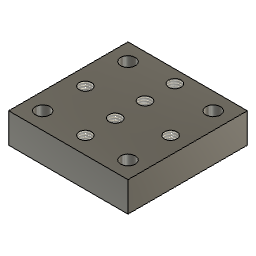
Dilution Attachment 28x28mm v2 (Autodesk Fusion 360 design; units mm, degrees)
Autodesk Fusion 360 part; units mm, degrees
note: some values were not read from the file. Set by a fixed rule: the direction of a hole.
sketch "Sketch1" plane through (0, 0, 0) normal (0, 0, 1) x (1, 0, 0)
  line L0 (0, 28) -> (28, 28)
  line L1 (28, 28) -> (28, 0)
  line L2 (28, 0) -> (0, 0)
  line L3 (0, 0) -> (0, 28)
  dimension "d1" = 28
  dimension "d2" = 28
  dimension "d13" = 28
  dimension "d14" = 28
  constraint horizontal L0
  constraint vertical L1
  constraint horizontal L2
  constraint vertical L3
  measures "d1" distance of L0.start L0.end
  measures "d2" distance of L0.start L2.end
  measures "d13" distance of L0.end L1.end
  measures "d14" distance of L1.end L2.end
sketch "Sketch2" plane through (0, 0, 0) normal (0, 0, 1) x (1, 0, 0)
  circle A0 centre (4, 24) radius 1.5
  circle A1 centre (4, 4) radius 1.5
  circle A2 centre (24, 4) radius 1.5
  circle A3 centre (24, 24) radius 1.5
  circle A4 centre (4, 14) radius 1.5
  circle A5 centre (14, 25) radius 1.5
  circle A6 centre (14, 18) radius 1.5
  circle A7 centre (14, 4) radius 1.5
  circle A8 centre (24, 14) radius 1.5
  circle A9 centre (14, 11) radius 1.5
  dimension "d15" = 3
  dimension "d16" = 3
  dimension "d17" = 3
  dimension "d18" = 3
  dimension "d19" = 3
  dimension "d20" = 3
  dimension "d21" = 3
  dimension "d22" = 3
  dimension "d23" = 3
  dimension "d24" = 3
  dimension "d25" = 10
  dimension "d26" = 10
  dimension "d27" = 10
  dimension "d28" = 10
  dimension "d29" = 10
  dimension "d30" = 10
  dimension "d31" = 7
  dimension "d32" = 7
  dimension "d33" = 7
  measures "d15" diameter of A0
  measures "d16" diameter of A5
  measures "d17" diameter of A3
  measures "d18" diameter of A6
  measures "d19" diameter of A4
  measures "d20" diameter of A8
  measures "d21" diameter of A9
  measures "d22" diameter of A7
  measures "d23" diameter of A2
  measures "d24" diameter of A1
  measures "d25" distance of A0.centre A4.centre
  measures "d26" distance of A1.centre A4.centre
  measures "d27" distance of A1.centre A7.centre
  measures "d28" distance of A2.centre A7.centre
  measures "d29" distance of A2.centre A8.centre
  measures "d30" distance of A3.centre A8.centre
  measures "d31" distance of A5.centre A6.centre
  measures "d32" distance of A6.centre A9.centre
  measures "d33" distance of A7.centre A9.centre
extrude "Extrude1" add sketch "Sketch1" along normal blind 7
hole "Hole1" at (14, 25, 0) at (4, 14, 0) at (14, 18, 0) at (14, 11, 0) at (24, 14, 0) at (14, 4, 0) direction (0, 0, 1) diameter 2.93 depth 7 tip angle 180
thread "Thread1" "ISO Metric profile 3.5 M3.5x0.6 6H" thread offset 0 thread depth 7.4
sketch "Sketch3" plane through (0, 0, 7) normal (0, 0, 1) x (-1, 0, 0)
  circle A0 centre (-24, -14) radius 1.465
  circle A1 centre (-14, -18) radius 1.465
  circle A2 centre (-14, -25) radius 1.465
  circle A3 centre (-4, -14) radius 1.465
  circle A4 centre (-14, -11) radius 1.465
  circle A5 centre (-14, -4) radius 1.465
  line L0 (0, 0) -> (-28, 0)
  line L1 (-28, 0) -> (-28, -28)
  line L2 (-28, -28) -> (0, -28)
  line L3 (0, -28) -> (0, 0)
  circle A6 centre (-4, -24) radius 2
  circle A7 centre (-4, -4) radius 2
  circle A8 centre (-24, -4) radius 2
  circle A9 centre (-24, -24) radius 2
hole "Hole2" at (4, 24, 7) at (24, 24, 7) at (24, 4, 7) at (4, 4, 7) direction (0, 0, -1) diameter 3.4 depth 7 tip angle 180
